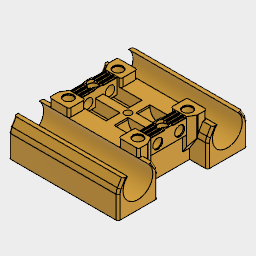
X_Carriage_F02 (Autodesk Fusion 360 design; units mm, degrees)
Autodesk Fusion 360 part; units mm, degrees
sketch "スケッチ1" plane through (0, 0, 0) normal (0, 0, 1) x (1, 0, 0)
  line L0 (-27.5, 32.5) -> (27.5, 32.5)
  line L1 (27.5, 32.5) -> (27.5, 12.5)
  line L2 (27.5, 12.5) -> (18.5, 12.5)
  line L3 (18.5, 12.5) -> (18.5, -12.5)
  line L4 (18.5, -12.5) -> (27.5, -12.5)
  line L5 (27.5, -12.5) -> (27.5, -32.5)
  line L6 (27.5, -32.5) -> (-27.5, -32.5)
  line L7 (-27.5, -32.5) -> (-27.5, -12.5)
  line L8 (-27.5, -12.5) -> (-18.5, -12.5)
  line L9 (-18.5, -12.5) -> (-18.5, 12.5)
  line L10 (-18.5, 12.5) -> (-27.5, 12.5)
  line L11 (-27.5, 12.5) -> (-27.5, 32.5)
  circle A0 centre (0, 0) radius 1.75
  dimension "d1" = 55
  dimension "d2" = 65
  dimension "d3" = 20
  dimension "d4" = 20
  dimension "d5" = 9
  dimension "d6" = 27.5
  dimension "d7" = 32.5
  dimension "d8" = 9
  dimension "d9" = 3.5
  measures "d1" distance of L5.end L6.end
  measures "d2" distance of L0 L6
  measures "d3" distance of L0.end L1.end
  measures "d4" distance of L4.end L5.end
  measures "d5" distance of L1.end L2.end
  measures "d6" distance of A0.centre L5
  measures "d7" distance of A0.centre L0
  measures "d8" distance of L9.end L10.end
  measures "d9" diameter of A0
extrude "押し出し1" add sketch "スケッチ1" along normal blind 17.3 makes body 1
sketch "スケッチ2" plane through (27.5, 0, 0) normal (1, 0, 0) x (0, 1, 0)
  line L0 (12.5, 0) -> (32.5, 0)
  line L1 (32.5, 0) -> (32.5, 17.3)
  line L2 (32.5, 17.3) -> (12.5, 17.3)
  line L3 (12.5, 17.3) -> (12.5, 0)
  line L4 (22.5, 0) -> (22.5, 17.3) construction
  line L5 (12.5, 12.6228) -> (32.5, 12.6228) construction
  circle A0 centre (22.5, 12) radius 7.495
  line L6 (32.5, 12.6228) -> (29.7996, 17.3)
  line L7 (32.5, 12.6228) -> (38.6199, 12.6228) construction
  line L8 (12.5, 12.6228) -> (15.2004, 17.3)
  line L9 (12.5, 17.3) -> (-12.5, 17.3)
  line L10 (0, 0) -> (0, 17.3) construction
  circle A1 centre (-22.5, 12) radius 7.495
  line L11 (-12.5, 12.6228) -> (-15.2004, 17.3)
  line L12 (-32.5, 12.6228) -> (-29.7996, 17.3)
  line L13 (-32.5, 17.3) -> (-12.5, 17.3)
  line L14 (-32.5, 0) -> (-32.5, 17.3)
  line L15 (-12.5, 17.3) -> (-12.5, 0)
  point P0 (0, 17.3)
  dimension "d12" = 12.6228
  dimension "d13" = 14.99
  dimension "d14" = 120
  dimension "d15" = 60
  dimension "d135" = 12
  measures "d12" distance of L0 L5
  measures "d13" diameter of A0
  measures "d14" angle of L6 L7
  measures "d15" angle of L7 L8
  measures "d135" distance of L4.start A0.centre
extrude "押し出し2" cut sketch "スケッチ2" against normal blind 55 contours L1 L2 L6 | L2 A0 | A1 L13 | L12 L13 L14 picked at (23.6851, 8.0373) picked at (-20.4164, 11.6826) bodies 1
extrude "押し出し3" cut sketch "スケッチ2" against normal blind 9 contours L2 L3 L8 | L11 L13 L15 bodies 1
extrude "押し出し4" cut sketch "スケッチ2" against normal blind 9 from surface at -46 contours L2 L3 L8 | L11 L13 L15 bodies 1
sketch "スケッチ3" plane through (0, 0, 17.3) normal (0, 0, 1) x (-1, 0, 0)
  line L0 (18.5, -15.2004) -> (18.5, 15.2004)
  line L1 (27.5, 15.2004) -> (27.5, 17.2005)
  line L2 (-27.5, 17.2005) -> (-27.5, 15.2004)
  line L3 (-18.5, 15.2004) -> (-18.5, -15.2004)
  line L4 (-18.5, -15.2004) -> (-27.5, -15.2004)
  line L5 (-27.5, -15.2004) -> (-27.5, -17.2005)
  line L6 (-27.5, -17.2005) -> (27.5, -17.2005)
  line L7 (27.5, -17.2005) -> (27.5, -15.2004)
  line L8 (27.5, -15.2004) -> (18.5, -15.2004)
  circle A0 centre (0, 0) radius 1.75
  line L9 (-12.5, -17.2005) -> (-12.5, -9)
  line L10 (-2, -9) -> (-22.5, -9)
  line L11 (-22.5, -9) -> (-22.5, -17.2005)
  line L12 (-22.5, -17.2005) -> (-12.5, -17.2005)
  line L13 (-2, -9) -> (-2, -2)
  line L14 (-2, -2) -> (-18.5, -2)
  line L15 (27.5, 17.2005) -> (-27.5, 17.2005)
  line L16 (-27.5, 15.2004) -> (-18.5, 15.2004)
  line L17 (18.5, 15.2004) -> (27.5, 15.2004)
  dimension "d23" = 10
  dimension "d24" = 12.5
  dimension "d26" = 7
  dimension "d27" = 2
  dimension "d28" = 16.5
  measures "d23" distance of L9.start L11.end
  measures "d24" distance of A0.centre L9.start
  measures "d26" distance of L13.end L10.start
  measures "d27" distance of A0.centre L14
  measures "d28" distance of L13.end L14.end
extrude "押し出し5" cut sketch "スケッチ3" against normal blind 5.9 contours L3 L10 L13 L14 bodies 1
fillet "フィレット3" radius 5 1 edges at (2, 5.5, 11.4) on bodies 1
mirror "ミラー1" about plane through (0, 0, 0) normal (0, 1, 0) of "押し出し5", "フィレット3"
mirror "ミラー2" about plane through (0, 0, 0) normal (1, 0, 0) of "押し出し5", "フィレット3", "ミラー1"
extrude "押し出し6" add sketch "スケッチ3" against normal blind 12.3 separate body contours L3 L4 L6 L9 L10 L11 L12 | L3 L4 L10 L11 makes body 2
chamfer "面取り2" distance 4 distance2 6.4 1 edges at (22.5, 13.1002, 5) measured on face at (17.8333, 13.8003, 5) on bodies 2
extrude "押し出し7" add sketch "スケッチ3" along normal blind 4.1 contours L3 L4 L6 L9 L10 L11 L12 | L3 L4 L10 L11 bodies 2
chamfer "面取り3" distance 2 distance2 3.5 1 edges at (22.5, 9, 16.4) measured on face at (15.8333, 9, 12.6) on bodies 2
sketch "スケッチ4" plane through (0, 0, 21.4) normal (0, 0, 1) x (-1, 0, 0)
  line L0 (-20.5, -9) -> (-22.5, -12.5)
  line L1 (-22.5, -12.5) -> (-22.5, -17.2005)
  line L2 (-22.5, -17.2005) -> (-12.5, -17.2005)
  line L3 (-12.5, -17.2005) -> (-12.5, -9)
  line L4 (-12.5, -9) -> (-20.5, -9)
  line L5 (-17.5, -9) -> (-17.5, -17.2005) construction
  line L6 (-22.5, -12.5) -> (-12.5, -12.5) construction
  circle A0 centre (-17.5, -12.5) radius 1.75
  circle A1 centre (-17.5, -12.5) radius 2.35
  circle A2 centre (-17.5, -12.5) radius 2.5
  dimension "d47" = 3.5
  dimension "d48" = 5
  dimension "d50" = 5
  dimension "d51" = 4.7
  dimension "d53" = 3.5
  measures "d47" distance of L3.end L6.end
  measures "d48" distance of L1 L5
  measures "d50" diameter of A2
  measures "d51" diameter of A1
  measures "d53" diameter of A0
fillet "フィレット1" radius 1 4 edges at (12.5, 9, 13.2) (12.5, 17.2005, 13.2) (22.5, 17.2005, 16.4) (22.5, 12.5, 16.4) on bodies 2
extrude "押し出し19" cut sketch "スケッチ2" against normal blind 20 contours L2 A0 picked at (23.6851, 8.0373) bodies 2
mirror "ミラー3" about plane through (0, 0, 0) normal (0, 1, 0) of bodies 2 makes body 3
sketch "スケッチ5" plane through (0, 9, 0) normal (0, -1, 0) x (1, 0, 0)
  line L0 (13.5, 21.4) -> (13.5, 5)
  line L1 (13.5, 5) -> (18.5, 5)
  line L2 (18.5, 5) -> (20.5, 8.2)
  line L3 (20.5, 8.2) -> (20.5, 21.4)
  line L4 (20.5, 21.4) -> (13.5, 21.4)
  line L5 (13.5, 13.4) -> (20.5, 13.4)
  line L6 (14.5, 13.4) -> (14.5, 21.4)
  line L7 (20.5, 20.95) -> (14.5, 20.95)
  line L8 (17.5, 20.95) -> (17.5, 20.2) construction
  arc A0 (17.0011, 20.5118) -> (17.9989, 20.5118) centre (17.5, 20.755) ccw
  arc A1 (16.9, 20.95) -> (17.0011, 20.5118) centre (17.9, 20.95) ccw
  arc A2 (17.9989, 20.5118) -> (18.1, 20.95) centre (17.1, 20.95) ccw
  arc A3 (15.9989, 20.5118) -> (16.1, 20.95) centre (15.1, 20.95) ccw
  arc A4 (15.0011, 20.5118) -> (15.9989, 20.5118) centre (15.5, 20.755) ccw
  arc A5 (14.9, 20.95) -> (15.0011, 20.5118) centre (15.9, 20.95) ccw
  arc A6 (19.9989, 20.5118) -> (20.1, 20.95) centre (19.1, 20.95) ccw
  arc A7 (19.0011, 20.5118) -> (19.9989, 20.5118) centre (19.5, 20.755) ccw
  arc A8 (18.9, 20.95) -> (19.0011, 20.5118) centre (19.9, 20.95) ccw
  dimension "d62" = 8
  dimension "d63" = 6
  dimension "d64" = 0.45
  dimension "d65" = 0.75
  dimension "d70" = 0.555
  dimension "d71" = 1
  dimension "d72" = 1
  dimension "d75" = 2
  dimension "d76" = 0
  measures "d62" distance of L4 L5
  measures "d63" distance of L3 L6
  measures "d64" distance of L4 L7
  measures "d65" distance of L8.start L8.end
  measures "d70" radius of A0
  measures "d71" radius of A1
  measures "d72" radius of A2
extrude "押し出し11" add sketch "スケッチ5" along normal up to surface (18 mm away) contours L3 L5 L6 L7 A0 A1 A2 A3 A4 A5 A6 A7 A8 bodies 2 3
fillet "フィレット2" radius 0.15 6 edges at (14.9, 0, 20.95) (16.1, 0, 20.95) (16.9, 0, 20.95) (18.1, 0, 20.95) (18.9, 0, 20.95) (20.1, 0, 20.95) on bodies 2
sketch "スケッチ6" plane through (0, 0, 13.4) normal (0, 0, -1) x (1, 0, 0)
  line L0 (20.5, 9) -> (14.5, 9)
  line L1 (14.5, 9) -> (14.5, -9)
  line L2 (14.5, -9) -> (20.5, -9)
  line L3 (20.5, -9) -> (20.5, 9)
  line L4 (14.5, 0) -> (20.5, 0) construction
  line L5 (14.5, 2) -> (20.5, 2)
  line L6 (14.5, -2) -> (20.5, -2)
  dimension "d87" = 2
  dimension "d88" = 2
  measures "d87" distance of L4 L5
  measures "d88" distance of L4 L6
extrude "押し出し15" add sketch "スケッチ6" against normal blind 8 contours L1 L3 L5 L6 bodies 2
sketch "スケッチ7" plane through (0, 0, 21.4) normal (0, 0, 1) x (-1, 0, 0)
  line L0 (-14.5, -2) -> (-14.5, 2)
  line L1 (-14.5, 2) -> (-20.5, 2)
  line L2 (-20.5, 2) -> (-20.5, -2)
  line L3 (-20.5, -2) -> (-14.5, -2)
  line L4 (-14.5, 0) -> (-20.5, 0) construction
  circle A0 centre (-17.5, 0) radius 1.75
  circle A1 centre (-17.5, 0) radius 2.35
  circle A2 centre (-17.5, 0) radius 2.5
  dimension "d91" = 3.5
  dimension "d92" = 4.7
  dimension "d93" = 5
  measures "d91" diameter of A0
  measures "d92" diameter of A1
  measures "d93" diameter of A2
sketch "スケッチ8" plane through (20.5, 0, 0) normal (1, 0, 0) x (0, 1, 0)
  line L0 (-9, 13.4) -> (9, 13.4)
  line L1 (9, 13.4) -> (9, 20.95)
  line L2 (9, 20.95) -> (2, 20.95)
  line L3 (2, 20.95) -> (2, 21.4)
  line L4 (2, 21.4) -> (-2, 21.4)
  line L5 (-2, 21.4) -> (-2, 20.95)
  line L6 (-2, 20.95) -> (-9, 20.95)
  line L7 (-9, 20.95) -> (-9, 13.4)
  line L8 (9, 16.9) -> (-9, 16.9) construction
  line L9 (5.5, 13.4) -> (5.5, 20.95) construction
  circle A0 centre (5.5, 16.9) radius 2.5
  circle A1 centre (5.5, 16.9) radius 2.35
  dimension "d104" = 3.5
  dimension "d105" = 3.5
  dimension "d106" = 5
  dimension "d107" = 4.7
  measures "d104" distance of L1 L9
  measures "d105" distance of L0 L8
  measures "d106" diameter of A0
  measures "d107" diameter of A1
extrude "押し出し20" cut sketch "スケッチ8" against normal blind 10 contours A1 bodies 2
extrude "押し出し21" cut sketch "スケッチ8" against normal blind 0.5 contours A0 bodies 2
mirror "ミラー6" about plane through (0, 0, 0) normal (0, 1, 0) of "押し出し20", "押し出し21"
mirror "ミラー5" about plane through (0, 0, 0) normal (1, 0, 0) of bodies 2 makes body 4
combine "結合1" operation add target body 1 tool bodies 2 4
sketch "スケッチ9" plane through (0, 0, 21.4) normal (0, 0, 1) x (-1, 0, 0)
  arc A0 (-22.3682, -12.2694) -> (-22.5, -12.7656) centre (-21.5, -12.7656) ccw
  line L0 (-22.5, -12.7656) -> (-22.5, -16.2005)
  arc A1 (-22.5, -16.2005) -> (-21.5, -17.2005) centre (-21.5, -16.2005) ccw
  line L1 (-21.5, -17.2005) -> (-13.5, -17.2005)
  arc A2 (-13.5, -17.2005) -> (-12.5, -16.2005) centre (-13.5, -16.2005) ccw
  line L2 (-12.5, -16.2005) -> (-12.5, -10)
  arc A3 (-12.5, -10) -> (-13.5, -9) centre (-13.5, -10) ccw
  line L3 (-13.5, -9) -> (-20.5, -9)
  line L4 (-20.5, -9) -> (-22.3682, -12.2694)
  line L5 (-12.5, -12.5) -> (-22.5, -12.5) construction
  line L6 (-17.5, -17.2005) -> (-17.5, -9.0071) construction
  circle A4 centre (-17.5, -12.5) radius 1.75
  circle A5 centre (-17.5, -12.5) radius 2.35
  circle A6 centre (-17.5, -12.5) radius 2.5
  dimension "d113" = 5
  dimension "d114" = 3.5
  dimension "d115" = 5
  dimension "d116" = 4.7
  dimension "d117" = 3.5
  measures "d113" distance of L2 L6
  measures "d114" distance of L3 L5
  measures "d115" diameter of A6
  measures "d116" diameter of A5
  measures "d117" diameter of A4
extrude "押し出し22" cut sketch "スケッチ9" against normal blind 14 contours A4 bodies 1
extrude "押し出し23" cut sketch "スケッチ9" against normal blind 5 contours A5 bodies 1
extrude "押し出し24" cut sketch "スケッチ9" against normal blind 0.5 contours A6 bodies 1
mirror "ミラー7" about plane through (0, 0, 0) normal (0, 1, 0) of "押し出し22", "押し出し23", "押し出し24"
mirror "ミラー8" about plane through (0, 0, 0) normal (1, 0, 0) of "押し出し22", "押し出し23", "押し出し24", "ミラー7"
extrude "押し出し25" cut sketch "スケッチ7" against normal blind 7.6 contours A0 bodies 1
extrude "押し出し26" cut sketch "スケッチ7" against normal blind 6 contours L3 A1 | L1 L3 A1 | L1 A1 bodies 1
extrude "押し出し27" cut sketch "スケッチ7" against normal blind 1.5 contours L3 A1 A2 | L1 L3 A1 A2 | L1 A1 A2 | L1 L3 A1 A2 bodies 1
mirror "ミラー9" about plane through (0, 0, 0) normal (1, 0, 0) of "押し出し25", "押し出し26", "押し出し27"
fillet "フィレット4" radius 5 6 edges at (0, 32.5, 12.6228) (24.982, 12.5, 12.6228) (-24.982, 12.5, 12.6228) (0, -32.5, 12.6228) (24.982, -12.5, 12.6228) (-24.982, -12.5, 12.6228) on bodies 1
fillet "フィレット5" radius 1 24 edges at (27.5, 12.5, 5.6415) (27.5, 12.6704, 12.5771) (27.5, 14.1851, 15.5415) (27.5, 32.5, 5.6415) (27.5, 32.3296, 12.5771) (27.5, 30.8149, 15.5415) (-27.5, 32.5, 5.6415) (-27.5, 32.3296, 12.5771) (-27.5, 30.8149, 15.5415) (-27.5, 12.5, 5.6415) (-27.5, 12.6704, 12.5771) (-27.5, 14.1851, 15.5415) (-27.5, -12.5, 5.6415) (-27.5, -12.6704, 12.5771) (-27.5, -14.1851, 15.5415) (-27.5, -32.5, 5.6415) (-27.5, -32.3296, 12.5771) (-27.5, -30.8149, 15.5415) (27.5, -32.5, 5.6415) (27.5, -32.3296, 12.5771) (27.5, -30.8149, 15.5415) (27.5, -12.5, 5.6415) (27.5, -12.6704, 12.5771) (27.5, -14.1851, 15.5415) on bodies 1
sketch "スケッチ10" plane through (0, 0, 0) normal (0, 0, -1) x (1, 0, 0)
  circle A0 centre (0, 0) radius 1.75
  arc A1 (26.5, 12.5) -> (27.5, 13.5) centre (26.5, 13.5) ccw
  line L0 (27.5, 13.5) -> (27.5, 31.5)
  arc A2 (27.5, 31.5) -> (26.5, 32.5) centre (26.5, 31.5) ccw
  line L1 (26.5, 32.5) -> (-26.5, 32.5)
  arc A3 (-26.5, 32.5) -> (-27.5, 31.5) centre (-26.5, 31.5) ccw
  line L2 (-27.5, 31.5) -> (-27.5, 13.5)
  arc A4 (-27.5, 13.5) -> (-26.5, 12.5) centre (-26.5, 13.5) ccw
  line L3 (-26.5, 12.5) -> (-18.5, 12.5)
  line L4 (-18.5, 12.5) -> (-18.5, -12.5)
  line L5 (-18.5, -12.5) -> (-26.5, -12.5)
  arc A5 (-26.5, -12.5) -> (-27.5, -13.5) centre (-26.5, -13.5) ccw
  line L6 (-27.5, -13.5) -> (-27.5, -31.5)
  arc A6 (-27.5, -31.5) -> (-26.5, -32.5) centre (-26.5, -31.5) ccw
  line L7 (-26.5, -32.5) -> (26.5, -32.5)
  arc A7 (26.5, -32.5) -> (27.5, -31.5) centre (26.5, -31.5) ccw
  line L8 (27.5, -31.5) -> (27.5, -13.5)
  arc A8 (27.5, -13.5) -> (26.5, -12.5) centre (26.5, -13.5) ccw
  line L9 (26.5, -12.5) -> (18.5, -12.5)
  line L10 (18.5, -12.5) -> (18.5, 12.5)
  line L11 (18.5, 12.5) -> (26.5, 12.5)
  circle A9 centre (12, 12) radius 1.525
  circle A10 centre (-12, 12) radius 1.525
  circle A11 centre (-12, -12) radius 1.525
  circle A12 centre (12, -12) radius 1.525
  dimension "d139" = 3.05
  dimension "d140" = 12
  dimension "d141" = 12
  dimension "d143" = 360
  measures "d139" diameter of A9
  measures "d140" distance of A0.centre A9.centre
  measures "d141" distance of A0.centre A9.centre
extrude "押し出し28" cut sketch "スケッチ10" against normal blind 10 contours A9 | A10 | A11 | A12 bodies 1
equation "d6 = d1 / 2"
equation "d7 = d2 / 2"
equation "d8 = d5"
